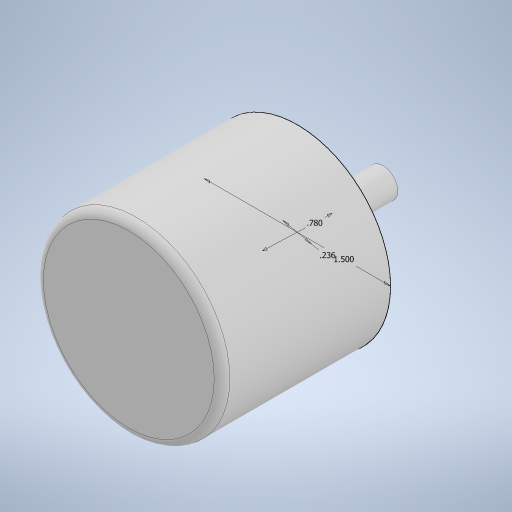
# Autodesk Inventor part: OpticalRotaryEncoder
Saved by Autodesk Inventor 2024 (Build 280153000, 153)
## iProperties
Created: 2025-01-04
Part Number: OpticalRotaryEncoder
Material: Generic
Document SubType Name: Modeling
Designer: Tommy Rohmann
Density: 1 g/cm^3
Appearance: Default
Author: Tommy Rohmann
Autodesk Inventor part; units mm, degrees
ref_plane "YZ Plane" through (0, 0, 0) normal (1, 0, 0) x (0, 1, 0)
ref_plane "XZ Plane" through (0, 0, 0) normal (0, 1, 0) x (-1, 0, 0)
ref_plane "XY Plane" through (0, 0, 0) normal (0, 0, 1) x (1, 0, 0)
sketch "Sketch1" plane through (0, 0, 0) normal (0, 0, 1) x (1, 0, 0)
  circle A0 centre (0, 0) radius 19.05
  circle A1 centre (0, 0) radius 9.906
  circle A2 centre (0, 0) radius 3
  dimension "d0" = 38.1
  dimension "d1" = 19.812
  dimension "d2" = 6
  constraints: 3 centre point, 3 coincident
  measures "d0" diameter of A0
  measures "d1" diameter of A1
  measures "d2" diameter of A2
extrude "Extrusion1" add sketch "Sketch1" along normal blind 34.417 contours A0 | A1 | A2
extrude "Extrusion2" add sketch "Sketch1" against normal blind 5.207 contours A1
extrude "Extrusion3" add sketch "Sketch1" against normal blind 17.5768 contours A2
fillet "Fillet1" radius 1.5875 1 edges at (-19.05, 0, 34.417)
body "Solid1"
